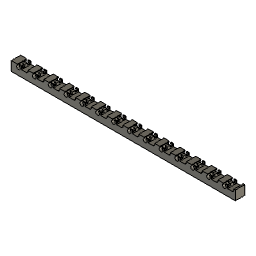
Assembly v11 (Autodesk Fusion 360 archive; units mm, degrees)
design "Pushing Bar"
Autodesk Fusion 360 part; units mm, degrees
sketch "Sketch1" plane through (0, 0, 0) normal (0, 0, 1) x (1, 0, 0)
  line L0 (390, 15) -> (-390, 15)
  line L1 (-390, 15) -> (-390, -15)
  line L2 (-390, -15) -> (390, -15)
  line L3 (390, -15) -> (390, 15)
  line L4 (390, 15) -> (-390, -15) construction
  line L5 (-390, 15) -> (390, -15) construction
  line L6 (3, -10) -> (-3, -10) construction
  line L7 (-3, -10) -> (-3, 10) construction
  line L8 (-3, 10) -> (3, 10) construction
  line L9 (3, 10) -> (3, -10) construction
  line L10 (3, -10) -> (-3, 10) construction
  line L11 (-3, -10) -> (3, 10) construction
  line L12 (-328.9372, 15) -> (390, 15)
  line L13 (390, 15) -> (390, -15)
  line L14 (390, -15) -> (-328.9372, -15)
  dimension "d2" = 780
  dimension "d5" = 20
  dimension "d6" = 6
  dimension "d7" = 5
  constraint horizontal L0
  constraint perpendicular L0 L1
  constraint parallel L0 L2
  constraint parallel L1 L3
  constraint coincident L4 origin
  constraint coincident L5 origin
  constraint horizontal L6
  constraint perpendicular L6 L7
  constraint parallel L6 L8
  constraint parallel L7 L9
  constraint coincident L10 origin
  constraint coincident L11 origin
  constraint horizontal L12
  constraint vertical L13
  constraint horizontal L14
  constraint coincident L0 L12.start
  measures "d2" distance of L0.start L0.end
  measures "d5" distance of L6.start L8.end
  measures "d6" distance of L7.end L8.end
  measures "d7" distance of L2 L6
extrude "Extrude1" add sketch "Sketch1" along normal mid plane 30
sketch "Sketch2" plane through (0, 0, 0) normal (0, 1, 0) x (1, 0, 0)
  circle A0 centre (339.2, -7.6834) radius 6 construction
  circle A1 centre (339.2, -11) radius 5
  line L0 (-390, -15) -> (390, -15)
  line L1 (334.2, -11) -> (344.2, -11) construction
  line L2 (390, -15) -> (390, 15) construction
  line L3 (342.2, -15) -> (336.2, -15)
  line L4 (336.2, -15) -> (336.2, -7)
  line L5 (336.2, -7) -> (342.2, -7)
  line L6 (342.2, -7) -> (342.2, -15)
  circle A2 centre (288.4, -11) radius 5
  circle A3 centre (237.6, -11) radius 5
  circle A4 centre (186.8, -11) radius 5
  circle A5 centre (136, -11) radius 5
  circle A6 centre (85.2, -11) radius 5
  circle A7 centre (34.4, -11) radius 5
  circle A8 centre (-16.4, -11) radius 5
  circle A9 centre (-67.2, -11) radius 5
  circle A10 centre (-118, -11) radius 5
  circle A11 centre (-168.8, -11) radius 5
  circle A12 centre (-219.6, -11) radius 5
  circle A13 centre (-270.4, -11) radius 5
  circle A14 centre (-321.2, -11) radius 5
  circle A15 centre (339.2, -12.3542) radius 4 construction
  dimension "d8" = 10
  dimension "d9" = 12
  dimension "d11" = 50.8
  dimension "d15" = 6
  dimension "d18" = -50.8
  dimension "d19" = 0
  dimension "d24" = 8
  constraint vertical A0.centre A1.centre
  constraint coincident A1 L1.start
  constraint coincident A1 L1.end
  constraint parallel L0 L1
  constraint coincident A1.centre L1
  constraint coincident A0 L1.start
  constraint horizontal L3
  constraint vertical L4
  constraint horizontal L5
  constraint vertical L6
  constraint coincident A1 L3.start
  constraint coincident L0 L3.start
  constraint coincident A1 L3.end
  constraint coincident A1 L5.end
  constraint coincident L3.end A15
  constraint coincident L3.start A15
  measures "d8" diameter of A1
  measures "d9" diameter of A0
  measures "d11" distance of A1.centre L2
  measures "d15" distance of L3.start L3.end
  measures "d24" diameter of A15
extrude "Extrude2" cut sketch "Sketch2" along normal mid plane 24 contours A1 L6 | A1 L5 | L0 L3 L4 L5 L6 | A1 L4 | L0 A14 | L0 A13 | L0 A12 | L0 A11 | L0 A10 | L0 A9 | L0 A8 | L0 A7 | L0 A6 | L0 A5 | L0 A4 | L0 A3 | L0 A2 picked at (-320.0174, -13.3398) picked at (-269.2174, -13.3398) picked at (-221.1787, -11.1742) picked at (-170.3787, -11.1742) picked at (-117.987, -11.8527) picked at (-66.8785, -11.7945) picked at (-17.7203, -12.3275) picked at (34.413, -11.8527) picked at (85.213, -11.8527) picked at (134.3807, -11.852) picked at (187.7455, -8.0418) picked at (238.5455, -8.0418) picked at (289.5826, -13.3398)
sketch "Sketch3" plane through (0, 0, 0) normal (0, 1, 0) x (1, 0, 0)
  circle A0 centre (339.2, -7.6834) radius 6
  line L0 (336.2, -15) -> (342.2, -15)
  line L1 (342.2, -12.8795) -> (342.2, -2.4872) construction
  line L2 (342.2, -2.4872) -> (336.2, -2.4872) construction
  line L3 (336.2, -2.4872) -> (336.2, -12.8795) construction
  circle A1 centre (339.2, -11) radius 5 construction
  line L4 (-390, -15) -> (390, -15)
  line L5 (342.2, -15) -> (342.2, -12.8795)
  line L6 (336.2, -12.8795) -> (336.2, -15)
  arc A2 (342.2, -12.8795) -> (336.2, -12.8795) centre (339.2, -7.6834) ccw
  arc A3 (336.2, -12.8795) -> (342.2, -12.8795) centre (339.2, -7.6834) ccw construction
  line L7 (285.4, -12.8795) -> (285.4, -15)
  line L8 (285.4, -15) -> (291.4, -15)
  arc A4 (291.4, -12.8795) -> (285.4, -12.8795) centre (288.4, -7.6834) ccw
  line L9 (291.4, -15) -> (291.4, -12.8795)
  line L10 (234.6, -12.8795) -> (234.6, -15)
  line L11 (234.6, -15) -> (240.6, -15)
  arc A5 (240.6, -12.8795) -> (234.6, -12.8795) centre (237.6, -7.6834) ccw
  line L12 (240.6, -15) -> (240.6, -12.8795)
  line L13 (183.8, -12.8795) -> (183.8, -15)
  line L14 (183.8, -15) -> (189.8, -15)
  arc A6 (189.8, -12.8795) -> (183.8, -12.8795) centre (186.8, -7.6834) ccw
  line L15 (189.8, -15) -> (189.8, -12.8795)
  line L16 (133, -12.8795) -> (133, -15)
  line L17 (133, -15) -> (139, -15)
  arc A7 (139, -12.8795) -> (133, -12.8795) centre (136, -7.6834) ccw
  line L18 (139, -15) -> (139, -12.8795)
  line L19 (82.2, -12.8795) -> (82.2, -15)
  line L20 (82.2, -15) -> (88.2, -15)
  arc A8 (88.2, -12.8795) -> (82.2, -12.8795) centre (85.2, -7.6834) ccw
  line L21 (88.2, -15) -> (88.2, -12.8795)
  line L22 (31.4, -12.8795) -> (31.4, -15)
  line L23 (31.4, -15) -> (37.4, -15)
  arc A9 (37.4, -12.8795) -> (31.4, -12.8795) centre (34.4, -7.6834) ccw
  line L24 (37.4, -15) -> (37.4, -12.8795)
  line L25 (-19.4, -12.8795) -> (-19.4, -15)
  line L26 (-19.4, -15) -> (-13.4, -15)
  arc A10 (-13.4, -12.8795) -> (-19.4, -12.8795) centre (-16.4, -7.6834) ccw
  line L27 (-13.4, -15) -> (-13.4, -12.8795)
  line L28 (-70.2, -12.8795) -> (-70.2, -15)
  line L29 (-70.2, -15) -> (-64.2, -15)
  arc A11 (-64.2, -12.8795) -> (-70.2, -12.8795) centre (-67.2, -7.6834) ccw
  line L30 (-64.2, -15) -> (-64.2, -12.8795)
  line L31 (-121, -12.8795) -> (-121, -15)
  line L32 (-121, -15) -> (-115, -15)
  arc A12 (-115, -12.8795) -> (-121, -12.8795) centre (-118, -7.6834) ccw
  line L33 (-115, -15) -> (-115, -12.8795)
  line L34 (-171.8, -12.8795) -> (-171.8, -15)
  line L35 (-171.8, -15) -> (-165.8, -15)
  arc A13 (-165.8, -12.8795) -> (-171.8, -12.8795) centre (-168.8, -7.6834) ccw
  line L36 (-165.8, -15) -> (-165.8, -12.8795)
  line L37 (-222.6, -12.8795) -> (-222.6, -15)
  line L38 (-222.6, -15) -> (-216.6, -15)
  arc A14 (-216.6, -12.8795) -> (-222.6, -12.8795) centre (-219.6, -7.6834) ccw
  line L39 (-216.6, -15) -> (-216.6, -12.8795)
  line L40 (-273.4, -12.8795) -> (-273.4, -15)
  line L41 (-273.4, -15) -> (-267.4, -15)
  arc A15 (-267.4, -12.8795) -> (-273.4, -12.8795) centre (-270.4, -7.6834) ccw
  line L42 (-267.4, -15) -> (-267.4, -12.8795)
  line L43 (-324.2, -12.8795) -> (-324.2, -15)
  line L44 (-324.2, -15) -> (-318.2, -15)
  arc A16 (-318.2, -12.8795) -> (-324.2, -12.8795) centre (-321.2, -7.6834) ccw
  line L45 (-318.2, -15) -> (-318.2, -12.8795)
  dimension "d22" = -50.8
  dimension "d23" = 0
  constraint equal A0 A2
  constraint horizontal L0
  constraint vertical L1
  constraint horizontal L2
  constraint vertical L3
  constraint coincident L0.start A1
  constraint coincident L0.end A1
  constraint coincident L0.end L4
  constraint coincident L2.end A2
  constraint coincident A0.centre A2.centre
  constraint vertical L5
  constraint vertical L6
  constraint concentric A2 A3
extrude "Extrude3" cut sketch "Sketch3" along normal through all and the other way through all
sketch "Sketch4" plane through (0, 0, 0) normal (0, 1, 0) x (1, 0, 0)
  line L0 (339.2, -9.5) -> (341.7981, -9.5) construction
  line L1 (349.2, -9.5) -> (349.2, -12.5) construction
  line L2 (341.7981, -12.5) -> (339.2, -12.5) construction
  line L3 (339.2, -12.5) -> (339.2, -9.5) construction
  line L4 (349.2, -6) -> (364.819, -6)
  line L5 (364.819, -6) -> (364.819, -16) construction
  line L6 (364.819, -16) -> (341.7981, -16)
  line L7 (349.2, -12.5) -> (349.2, -9.5) construction
  line L8 (349.2, -9.5) -> (349.2, -6)
  arc A0 (364.819, -16) -> (364.819, -6) centre (364.819, -11) ccw
  arc A1 (364.819, -6) -> (364.819, -16) centre (364.819, -11) ccw construction
  line L9 (341.7981, -9.5) -> (349.2, -9.5)
  arc A2 (341.7981, -9.5) -> (341.7981, -12.5) centre (339.2, -11) ccw construction
  line L10 (341.7981, -16) -> (341.7981, -9.5)
  line L11 (349.2, -6) -> (364.819, -6)
  line L12 (364.819, -16) -> (349.2, -16)
  line L13 (349.2, -16) -> (349.2, -6)
  line L14 (349.2, -16) -> (349.2, -6)
  arc A3 (314.019, -16) -> (314.019, -6) centre (314.019, -11) ccw
  line L15 (314.019, -16) -> (298.4, -16)
  line L16 (314.019, -16) -> (290.9981, -16)
  line L17 (290.9981, -16) -> (290.9981, -9.5)
  line L18 (290.9981, -9.5) -> (298.4, -9.5)
  line L19 (298.4, -9.5) -> (298.4, -6)
  line L20 (298.4, -6) -> (314.019, -6)
  arc A4 (263.219, -16) -> (263.219, -6) centre (263.219, -11) ccw
  line L21 (263.219, -16) -> (247.6, -16)
  line L22 (263.219, -16) -> (240.1981, -16)
  line L23 (240.1981, -16) -> (240.1981, -9.5)
  line L24 (240.1981, -9.5) -> (247.6, -9.5)
  line L25 (247.6, -9.5) -> (247.6, -6)
  line L26 (247.6, -6) -> (263.219, -6)
  arc A5 (212.419, -16) -> (212.419, -6) centre (212.419, -11) ccw
  line L27 (212.419, -16) -> (196.8, -16)
  line L28 (212.419, -16) -> (189.3981, -16)
  line L29 (189.3981, -16) -> (189.3981, -9.5)
  line L30 (189.3981, -9.5) -> (196.8, -9.5)
  line L31 (196.8, -9.5) -> (196.8, -6)
  line L32 (196.8, -6) -> (212.419, -6)
  arc A6 (161.619, -16) -> (161.619, -6) centre (161.619, -11) ccw
  line L33 (161.619, -16) -> (146, -16)
  line L34 (161.619, -16) -> (138.5981, -16)
  line L35 (138.5981, -16) -> (138.5981, -9.5)
  line L36 (138.5981, -9.5) -> (146, -9.5)
  line L37 (146, -9.5) -> (146, -6)
  line L38 (146, -6) -> (161.619, -6)
  arc A7 (110.819, -16) -> (110.819, -6) centre (110.819, -11) ccw
  line L39 (110.819, -16) -> (95.2, -16)
  line L40 (110.819, -16) -> (87.7981, -16)
  line L41 (87.7981, -16) -> (87.7981, -9.5)
  line L42 (87.7981, -9.5) -> (95.2, -9.5)
  line L43 (95.2, -9.5) -> (95.2, -6)
  line L44 (95.2, -6) -> (110.819, -6)
  arc A8 (60.019, -16) -> (60.019, -6) centre (60.019, -11) ccw
  line L45 (60.019, -16) -> (44.4, -16)
  line L46 (60.019, -16) -> (36.9981, -16)
  line L47 (36.9981, -16) -> (36.9981, -9.5)
  line L48 (36.9981, -9.5) -> (44.4, -9.5)
  line L49 (44.4, -9.5) -> (44.4, -6)
  line L50 (44.4, -6) -> (60.019, -6)
  arc A9 (9.219, -16) -> (9.219, -6) centre (9.219, -11) ccw
  line L51 (9.219, -16) -> (-6.4, -16)
  line L52 (9.219, -16) -> (-13.8019, -16)
  line L53 (-13.8019, -16) -> (-13.8019, -9.5)
  line L54 (-13.8019, -9.5) -> (-6.4, -9.5)
  line L55 (-6.4, -9.5) -> (-6.4, -6)
  line L56 (-6.4, -6) -> (9.219, -6)
  arc A10 (-41.581, -16) -> (-41.581, -6) centre (-41.581, -11) ccw
  line L57 (-41.581, -16) -> (-57.2, -16)
  line L58 (-41.581, -16) -> (-64.6019, -16)
  line L59 (-64.6019, -16) -> (-64.6019, -9.5)
  line L60 (-64.6019, -9.5) -> (-57.2, -9.5)
  line L61 (-57.2, -9.5) -> (-57.2, -6)
  line L62 (-57.2, -6) -> (-41.581, -6)
  arc A11 (-92.381, -16) -> (-92.381, -6) centre (-92.381, -11) ccw
  line L63 (-92.381, -16) -> (-108, -16)
  line L64 (-92.381, -16) -> (-115.4019, -16)
  line L65 (-115.4019, -16) -> (-115.4019, -9.5)
  line L66 (-115.4019, -9.5) -> (-108, -9.5)
  line L67 (-108, -9.5) -> (-108, -6)
  line L68 (-108, -6) -> (-92.381, -6)
  arc A12 (-143.181, -16) -> (-143.181, -6) centre (-143.181, -11) ccw
  line L69 (-143.181, -16) -> (-158.8, -16)
  line L70 (-143.181, -16) -> (-166.2019, -16)
  line L71 (-166.2019, -16) -> (-166.2019, -9.5)
  line L72 (-166.2019, -9.5) -> (-158.8, -9.5)
  line L73 (-158.8, -9.5) -> (-158.8, -6)
  line L74 (-158.8, -6) -> (-143.181, -6)
  arc A13 (-193.981, -16) -> (-193.981, -6) centre (-193.981, -11) ccw
  line L75 (-193.981, -16) -> (-209.6, -16)
  line L76 (-193.981, -16) -> (-217.0019, -16)
  line L77 (-217.0019, -16) -> (-217.0019, -9.5)
  line L78 (-217.0019, -9.5) -> (-209.6, -9.5)
  line L79 (-209.6, -9.5) -> (-209.6, -6)
  line L80 (-209.6, -6) -> (-193.981, -6)
  arc A14 (-244.781, -16) -> (-244.781, -6) centre (-244.781, -11) ccw
  line L81 (-244.781, -16) -> (-260.4, -16)
  line L82 (-244.781, -16) -> (-267.8019, -16)
  line L83 (-267.8019, -16) -> (-267.8019, -9.5)
  line L84 (-267.8019, -9.5) -> (-260.4, -9.5)
  line L85 (-260.4, -9.5) -> (-260.4, -6)
  line L86 (-260.4, -6) -> (-244.781, -6)
  arc A15 (-295.581, -16) -> (-295.581, -6) centre (-295.581, -11) ccw
  line L87 (-295.581, -16) -> (-311.2, -16)
  line L88 (-295.581, -16) -> (-318.6019, -16)
  line L89 (-318.6019, -16) -> (-318.6019, -9.5)
  line L90 (-318.6019, -9.5) -> (-311.2, -9.5)
  line L91 (-311.2, -9.5) -> (-311.2, -6)
  line L92 (-311.2, -6) -> (-295.581, -6)
  point P0 (339.2, -11)
  point P1 (349.2, -11)
  dimension "d25" = 6
  dimension "d26" = 3
  dimension "d27" = 10
  dimension "d29" = 15.619
  dimension "d31" = 3.5
  dimension "d32" = 5
  dimension "d43" = -50.8
  dimension "d44" = 0
  constraint coincident P0 A2.centre
  constraint horizontal L0
  constraint vertical L1
  constraint horizontal L2
  constraint vertical L3
  constraint coincident P0 L3
  constraint midpoint P0 L3
  constraint horizontal L4
  constraint vertical L5
  constraint horizontal L6
  constraint vertical L7
  constraint collinear L1 L7
  constraint coincident L7 P1
  constraint midpoint L1 P1
  constraint midpoint L5 A0.centre
  constraint concentric A0 A1
  constraint horizontal L9
  constraint vertical L8
  constraint vertical L10
  constraint horizontal L11
  constraint horizontal L12
  constraint vertical L13
  constraint vertical L14
  measures "d25" diameter of A2
  measures "d26" distance of L0 L2
  measures "d27" distance of P0 L1
  measures "d29" distance of L4.start L4.end
  measures "d31" distance of L1.start L4.start
  measures "d32" radius of A1
extrude "Extrude4" cut sketch "Sketch4" along normal blind 7 from surface at 5
extrude "Extrude5" cut sketch "Sketch4" against normal blind 7 from surface at -5
extrude "Extrude6" cut sketch "Sketch4" along normal through all and the other way through all contours L4 L6 L8 A0 L11 L12 L13 L14
sketch "Sketch5" plane through (0, 0, 0) normal (0, 1, 0) x (1, 0, 0)
  line L0 (349.2, -16) -> (369.819, -16)
  line L1 (369.819, -16) -> (369.819, -11)
  line L2 (364.819, -6) -> (349.2, -6)
  line L3 (349.2, -6) -> (349.2, -16)
  arc A0 (364.819, -16) -> (364.819, -6) centre (364.819, -11) ccw
  arc A1 (369.819, -11) -> (364.819, -6) centre (364.819, -11) ccw
  line L4 (369.819, -6) -> (364.819, -6) construction
  line L5 (369.819, -11) -> (369.819, -6) construction
  line L6 (298.4, -16) -> (319.019, -16)
  line L7 (298.4, -6) -> (298.4, -16)
  line L8 (314.019, -6) -> (298.4, -6)
  arc A2 (319.019, -11) -> (314.019, -6) centre (314.019, -11) ccw
  line L9 (319.019, -16) -> (319.019, -11)
  line L10 (247.6, -16) -> (268.219, -16)
  line L11 (247.6, -6) -> (247.6, -16)
  line L12 (263.219, -6) -> (247.6, -6)
  arc A3 (268.219, -11) -> (263.219, -6) centre (263.219, -11) ccw
  line L13 (268.219, -16) -> (268.219, -11)
  line L14 (196.8, -16) -> (217.419, -16)
  line L15 (196.8, -6) -> (196.8, -16)
  line L16 (212.419, -6) -> (196.8, -6)
  arc A4 (217.419, -11) -> (212.419, -6) centre (212.419, -11) ccw
  line L17 (217.419, -16) -> (217.419, -11)
  line L18 (146, -16) -> (166.619, -16)
  line L19 (146, -6) -> (146, -16)
  line L20 (161.619, -6) -> (146, -6)
  arc A5 (166.619, -11) -> (161.619, -6) centre (161.619, -11) ccw
  line L21 (166.619, -16) -> (166.619, -11)
  line L22 (95.2, -16) -> (115.819, -16)
  line L23 (95.2, -6) -> (95.2, -16)
  line L24 (110.819, -6) -> (95.2, -6)
  arc A6 (115.819, -11) -> (110.819, -6) centre (110.819, -11) ccw
  line L25 (115.819, -16) -> (115.819, -11)
  line L26 (44.4, -16) -> (65.019, -16)
  line L27 (44.4, -6) -> (44.4, -16)
  line L28 (60.019, -6) -> (44.4, -6)
  arc A7 (65.019, -11) -> (60.019, -6) centre (60.019, -11) ccw
  line L29 (65.019, -16) -> (65.019, -11)
  line L30 (-6.4, -16) -> (14.219, -16)
  line L31 (-6.4, -6) -> (-6.4, -16)
  line L32 (9.219, -6) -> (-6.4, -6)
  arc A8 (14.219, -11) -> (9.219, -6) centre (9.219, -11) ccw
  line L33 (14.219, -16) -> (14.219, -11)
  line L34 (-57.2, -16) -> (-36.581, -16)
  line L35 (-57.2, -6) -> (-57.2, -16)
  line L36 (-41.581, -6) -> (-57.2, -6)
  arc A9 (-36.581, -11) -> (-41.581, -6) centre (-41.581, -11) ccw
  line L37 (-36.581, -16) -> (-36.581, -11)
  line L38 (-108, -16) -> (-87.381, -16)
  line L39 (-108, -6) -> (-108, -16)
  line L40 (-92.381, -6) -> (-108, -6)
  arc A10 (-87.381, -11) -> (-92.381, -6) centre (-92.381, -11) ccw
  line L41 (-87.381, -16) -> (-87.381, -11)
  line L42 (-158.8, -16) -> (-138.181, -16)
  line L43 (-158.8, -6) -> (-158.8, -16)
  line L44 (-143.181, -6) -> (-158.8, -6)
  arc A11 (-138.181, -11) -> (-143.181, -6) centre (-143.181, -11) ccw
  line L45 (-138.181, -16) -> (-138.181, -11)
  line L46 (-209.6, -16) -> (-188.981, -16)
  line L47 (-209.6, -6) -> (-209.6, -16)
  line L48 (-193.981, -6) -> (-209.6, -6)
  arc A12 (-188.981, -11) -> (-193.981, -6) centre (-193.981, -11) ccw
  line L49 (-188.981, -16) -> (-188.981, -11)
  line L50 (-260.4, -16) -> (-239.781, -16)
  line L51 (-260.4, -6) -> (-260.4, -16)
  line L52 (-244.781, -6) -> (-260.4, -6)
  arc A13 (-239.781, -11) -> (-244.781, -6) centre (-244.781, -11) ccw
  line L53 (-239.781, -16) -> (-239.781, -11)
  line L54 (-311.2, -16) -> (-290.581, -16)
  line L55 (-311.2, -6) -> (-311.2, -16)
  line L56 (-295.581, -6) -> (-311.2, -6)
  arc A14 (-290.581, -11) -> (-295.581, -6) centre (-295.581, -11) ccw
  line L57 (-290.581, -16) -> (-290.581, -11)
  point P0 (349.2, -16)
  dimension "d47" = -50.8
  dimension "d48" = 0
  constraint horizontal L0
  constraint vertical L1
  constraint horizontal L2
  constraint vertical L3
  constraint tangent L1 A0
  constraint tangent L0 A0
  constraint tangent L2 A0
  constraint coincident L3 P0
  constraint coincident L2.start A0.end
  constraint midpoint A0 L1.end
extrude "Extrude7" cut sketch "Sketch5" along normal through all and the other way through all
sketch "Sketch6" plane through (0, 0, 15) normal (0, 0, 1) x (-1, 0, 0)
  line L0 (324.2, 15) -> (324.2, 12)
  line L1 (324.2, 12) -> (324.2, -12)
  line L2 (324.2, -12) -> (324.2, -15)
  line L3 (324.2, -15) -> (390, -15)
  line L4 (390, -15) -> (390, 15)
  line L5 (390, 15) -> (324.2, 15)
  line L6 (390, 15) -> (344.2, 15)
  line L7 (344.2, 15) -> (344.2, -15)
  line L8 (344.2, -15) -> (390, -15)
  line L9 (390, -15) -> (390, 15)
  line L10 (-390, -15) -> (-374.819, -15)
  line L11 (-374.819, -15) -> (-374.819, 15)
  line L12 (-374.819, 15) -> (-390, 15)
  line L13 (-390, 15) -> (-390, -15)
  line L14 (-390, -15) -> (-369.819, -15)
  line L15 (-369.819, 15) -> (-390, 15)
  line L16 (-390, 15) -> (-390, -15)
  line L17 (-369.819, -15) -> (-369.819, 15)
  dimension "d50" = 20
  dimension "d52" = 5
  constraint horizontal L6
  constraint vertical L7
  constraint horizontal L8
  constraint vertical L9
  constraint coincident L3 L7.end
  constraint coincident L4.end L5.start
  constraint horizontal L10
  constraint vertical L11
  constraint horizontal L12
  constraint vertical L13
  constraint collinear L10 L14
  constraint collinear L12 L15
  constraint collinear L13 L16
  measures "d50" distance of L1 L7
  measures "d52" distance of L11 L17
extrude "Extrude8" cut sketch "Sketch6" against normal through all contours L3 L4 L5 L6 L7 L8 L9 | L10 L11 L12 L13 L14 L15 L16
equation "d8 = 8 mm + 2 mm"
equation "d11 = ( 25.4 * 2 ) * 1 mm"
equation "d18 = ( -25.4 * 2 ) * 1 mm"
equation "d43 = ( -25.4 * 2 ) * 1 mm"
equation "d47 = ( -25.4 * 2 ) * 1 mm"

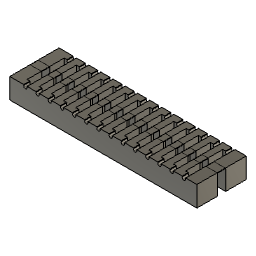
design "Grate Bars"
Autodesk Fusion 360 part; units mm, degrees
sketch "Sketch1" plane through (0, 0, 0) normal (0, 0, 1) x (1, 0, 0)
  line L0 (390, -102.9) -> (-390, -102.9)
  line L1 (-390, -102.9) -> (-390, 102.9)
  line L2 (-390, 102.9) -> (390, 102.9)
  line L3 (390, 102.9) -> (390, -102.9)
  line L4 (390, -102.9) -> (-390, 102.9) construction
  line L5 (-390, -102.9) -> (390, 102.9) construction
  dimension "d1" = 780
  dimension "d2" = 205.8
  constraint horizontal L0
  constraint perpendicular L0 L1
  constraint parallel L0 L2
  constraint parallel L1 L3
  constraint coincident L4 origin
  constraint coincident L5 origin
  measures "d1" distance of L1.end L2.end
  measures "d2" distance of L0.start L2.end
extrude "Extrude1" add sketch "Sketch1" along normal mid plane 85
sketch "Sketch2" plane through (0, 0, 42.5) normal (0, 0, 1) x (-1, 0, 0)
  line L0 (-390, -102.9) -> (390, -102.9)
  line L1 (390, -102.9) -> (390, 102.9)
  line L2 (390, 102.9) -> (-390, 102.9)
  line L3 (-390, 102.9) -> (-390, -102.9)
  line L4 (317.5, 77.5) -> (342.9, 77.5)
  line L5 (342.9, 77.5) -> (342.9, -77.5)
  line L6 (342.9, -77.5) -> (317.5, -77.5)
  line L7 (317.5, -77.5) -> (317.5, 77.5)
  line L8 (317.5, 77.5) -> (342.9, -77.5) construction
  line L9 (342.9, 77.5) -> (317.5, -77.5) construction
  line L10 (292.1, 77.5) -> (292.1, -77.5)
  line L11 (292.1, -77.5) -> (266.7, -77.5)
  line L12 (266.7, -77.5) -> (266.7, 77.5)
  line L13 (266.7, 77.5) -> (292.1, 77.5)
  line L14 (241.3, 77.5) -> (241.3, -77.5)
  line L15 (241.3, -77.5) -> (215.9, -77.5)
  line L16 (215.9, -77.5) -> (215.9, 77.5)
  line L17 (215.9, 77.5) -> (241.3, 77.5)
  line L18 (190.5, 77.5) -> (190.5, -77.5)
  line L19 (190.5, -77.5) -> (165.1, -77.5)
  line L20 (165.1, -77.5) -> (165.1, 77.5)
  line L21 (165.1, 77.5) -> (190.5, 77.5)
  line L22 (139.7, 77.5) -> (139.7, -77.5)
  line L23 (139.7, -77.5) -> (114.3, -77.5)
  line L24 (114.3, -77.5) -> (114.3, 77.5)
  line L25 (114.3, 77.5) -> (139.7, 77.5)
  line L26 (88.9, 77.5) -> (88.9, -77.5)
  line L27 (88.9, -77.5) -> (63.5, -77.5)
  line L28 (63.5, -77.5) -> (63.5, 77.5)
  line L29 (63.5, 77.5) -> (88.9, 77.5)
  line L30 (38.1, 77.5) -> (38.1, -77.5)
  line L31 (38.1, -77.5) -> (12.7, -77.5)
  line L32 (12.7, -77.5) -> (12.7, 77.5)
  line L33 (12.7, 77.5) -> (38.1, 77.5)
  line L34 (-12.7, 77.5) -> (-12.7, -77.5)
  line L35 (-12.7, -77.5) -> (-38.1, -77.5)
  line L36 (-38.1, -77.5) -> (-38.1, 77.5)
  line L37 (-38.1, 77.5) -> (-12.7, 77.5)
  line L38 (-63.5, 77.5) -> (-63.5, -77.5)
  line L39 (-63.5, -77.5) -> (-88.9, -77.5)
  line L40 (-88.9, -77.5) -> (-88.9, 77.5)
  line L41 (-88.9, 77.5) -> (-63.5, 77.5)
  line L42 (-114.3, 77.5) -> (-114.3, -77.5)
  line L43 (-114.3, -77.5) -> (-139.7, -77.5)
  line L44 (-139.7, -77.5) -> (-139.7, 77.5)
  line L45 (-139.7, 77.5) -> (-114.3, 77.5)
  line L46 (-165.1, 77.5) -> (-165.1, -77.5)
  line L47 (-165.1, -77.5) -> (-190.5, -77.5)
  line L48 (-190.5, -77.5) -> (-190.5, 77.5)
  line L49 (-190.5, 77.5) -> (-165.1, 77.5)
  line L50 (-215.9, 77.5) -> (-215.9, -77.5)
  line L51 (-215.9, -77.5) -> (-241.3, -77.5)
  line L52 (-241.3, -77.5) -> (-241.3, 77.5)
  line L53 (-241.3, 77.5) -> (-215.9, 77.5)
  line L54 (-266.7, 77.5) -> (-266.7, -77.5)
  line L55 (-266.7, -77.5) -> (-292.1, -77.5)
  line L56 (-292.1, -77.5) -> (-292.1, 77.5)
  line L57 (-292.1, 77.5) -> (-266.7, 77.5)
  line L58 (-317.5, 77.5) -> (-317.5, -77.5)
  line L59 (-317.5, -77.5) -> (-342.9, -77.5)
  line L60 (-342.9, -77.5) -> (-342.9, 77.5)
  line L61 (-342.9, 77.5) -> (-317.5, 77.5)
  point P0 (330.2, 0)
  dimension "d5" = 25.4
  dimension "d7" = 25.4
  dimension "d10" = -50.8
  dimension "d11" = 0
  dimension "d14" = 47.1
  constraint horizontal L4
  constraint perpendicular L4 L5
  constraint parallel L4 L6
  constraint parallel L5 L7
  constraint coincident L8 P0
  constraint coincident L9 P0
  constraint horizontal origin P0
  measures "d5" distance of L0 L6
  measures "d7" distance of L4.start L4.end
  measures "d14" distance of L1 L5
extrude "Extrude2" cut sketch "Sketch2" against normal up to surface (85 mm away) contours L4 L5 L6 L7 | L10 L11 L12 L13 | L14 L15 L16 L17 | L18 L19 L20 L21 | L22 L23 L24 L25 | L26 L27 L28 L29 | L30 L31 L32 L33 | L34 L35 L36 L37 | L38 L39 L40 L41 | L42 L43 L44 L45 | L46 L47 L48 L49 | L50 L51 L52 L53 | L54 L55 L56 L57 | L58 L59 L60 L61
sketch "Sketch3" plane through (0, 0, 0) normal (0, 1, 0) x (1, 0, 0)
  circle A0 centre (335.9, -37.5) radius 7
  line L0 (317.5, -42.5) -> (317.5, 42.5)
  line L1 (390, -42.5) -> (-390, -42.5)
  line L2 (342.9, -42.5) -> (342.9, 42.5)
  circle A1 centre (285.1, -37.5) radius 7
  circle A2 centre (234.3, -37.5) radius 7
  circle A3 centre (183.5, -37.5) radius 7
  circle A4 centre (132.7, -37.5) radius 7
  circle A5 centre (81.9, -37.5) radius 7
  circle A6 centre (31.1, -37.5) radius 7
  circle A7 centre (-19.7, -37.5) radius 7
  circle A8 centre (-70.5, -37.5) radius 7
  circle A9 centre (-121.3, -37.5) radius 7
  circle A10 centre (-172.1, -37.5) radius 7
  circle A11 centre (-222.9, -37.5) radius 7
  circle A12 centre (-273.7, -37.5) radius 7
  circle A13 centre (-324.5, -37.5) radius 7
  dimension "d19" = 14
  dimension "d23" = 7
  dimension "d24" = 5
  dimension "d27" = -50.8
  dimension "d28" = 0
  measures "d19" diameter of A0
  measures "d23" distance of A0.centre L2
  measures "d24" distance of A0.centre L1
extrude "Extrude3" cut sketch "Sketch3" along normal through all and the other way through all contours A0 L1 | L1 A1 | L1 A2 | L1 A3 | L1 A4 | L1 A5 | L1 A6 | L1 A7 | L1 A8 | L1 A9 | L1 A10 | L1 A11 | L1 A12 | L1 A13 picked at (338.1343, -37.5876) picked at (287.3343, -37.5876) picked at (232.5837, -36.5434) picked at (181.7837, -36.5434) picked at (131.458, -35.7084) picked at (83.3358, -37.9253) picked at (29.0436, -38.7503) picked at (-18.0005, -40.5961) picked at (-69.9038, -38.5775) picked at (-120.1856, -37.8147) picked at (-170.3604, -35.9462) picked at (-220.8946, -36.7332) picked at (-271.4657, -37.5876) picked at (-322.2657, -37.5876)
fillet "Fillet1" radius 1 8 edges at (340.799, -90.2, 42.5) (331.001, -90.2, 42.5) (340.799, 90.2, 42.5) (331.001, 90.2, 42.5) (289.999, -90.2, 42.5) (280.201, -90.2, 42.5) (289.999, 90.2, 42.5) (280.201, 90.2, 42.5)
fillet "Fillet1" radius 1 48 edges at (229.401, 90.2, 42.5) (239.199, 90.2, 42.5) (229.401, -90.2, 42.5) (239.199, -90.2, 42.5) (188.399, -90.2, 42.5) (178.601, -90.2, 42.5) (188.399, 90.2, 42.5) (178.601, 90.2, 42.5) (137.599, 90.2, 42.5) (127.801, 90.2, 42.5) (137.599, -90.2, 42.5) (127.801, -90.2, 42.5) (86.799, -90.2, 42.5) (77.001, -90.2, 42.5) (86.799, 90.2, 42.5) (77.001, 90.2, 42.5) (35.999, 90.2, 42.5) (26.201, 90.2, 42.5) (35.999, -90.2, 42.5) (26.201, -90.2, 42.5) (-14.801, -90.2, 42.5) (-24.599, -90.2, 42.5) (-14.801, 90.2, 42.5) (-24.599, 90.2, 42.5) (-65.601, 90.2, 42.5) (-75.399, 90.2, 42.5) (-65.601, -90.2, 42.5) (-75.399, -90.2, 42.5) (-116.401, -90.2, 42.5) (-126.199, -90.2, 42.5) (-116.401, 90.2, 42.5) (-126.199, 90.2, 42.5) (-167.201, 90.2, 42.5) (-176.999, 90.2, 42.5) (-167.201, -90.2, 42.5) (-176.999, -90.2, 42.5) (-218.001, -90.2, 42.5) (-227.799, -90.2, 42.5) (-218.001, 90.2, 42.5) (-227.799, 90.2, 42.5) (-268.801, 90.2, 42.5) (-278.599, 90.2, 42.5) (-278.599, -90.2, 42.5) (-268.801, -90.2, 42.5) (-329.399, -90.2, 42.5) (-319.601, -90.2, 42.5) (-319.601, 90.2, 42.5) (-329.399, 90.2, 42.5)
sketch "Sketch4" plane through (390, 0, 0) normal (1, 0, 0) x (0, 1, 0)
  line L0 (102.9, -42.5) -> (102.9, 42.5)
  line L1 (102.9, 42.5) -> (-102.9, 42.5)
  line L2 (-102.9, 42.5) -> (-102.9, -42.5)
  line L3 (-102.9, -42.5) -> (102.9, -42.5)
  line L4 (-17, -42.5) -> (17, -42.5)
  line L5 (17, -42.5) -> (17, 40.5)
  line L6 (17, 40.5) -> (-17, 40.5)
  line L7 (-17, 40.5) -> (-17, -42.5)
  line L8 (-17, 40.5) -> (17, -42.5) construction
  line L9 (17, 40.5) -> (-17, -42.5) construction
  line L10 (0, 40.5) -> (0, -42.5) construction
  point P0 (0, -1)
  dimension "d34" = 17
  dimension "d36" = 2
  constraint horizontal L4
  constraint vertical L5
  constraint horizontal L6
  constraint vertical L7
  constraint coincident L3 L4.start
  constraint midpoint L9 P0
  constraint coincident L6 L10.start
  constraint coincident L3 L10.end
  constraint vertical L10
  constraint coincident origin L10
  constraint vertical origin P0
  measures "d34" distance of L7 L10
  measures "d36" distance of L1 L6
extrude "Extrude4" cut sketch "Sketch4" along normal through all and the other way through all contours L3 L4 L5 L6 L7
sketch "Sketch5" plane through (390, 0, 0) normal (1, 0, 0) x (0, 1, 0)
  line L0 (-17, -42.5) -> (-17, 40.5)
  line L1 (-17, 40.5) -> (17, 40.5)
  line L2 (17, 40.5) -> (17, -42.5)
  line L3 (17, -42.5) -> (102.9, -42.5)
  line L4 (102.9, -42.5) -> (102.9, 42.5)
  line L5 (102.9, 42.5) -> (-102.9, 42.5)
  line L6 (-102.9, 42.5) -> (-102.9, -42.5)
  line L7 (-102.9, -42.5) -> (-17, -42.5)
  line L8 (-21.5, 40.5) -> (21.5, 40.5)
  line L9 (21.5, 40.5) -> (21.5, -2.5)
  line L10 (21.5, -2.5) -> (-21.5, -2.5)
  line L11 (-21.5, -2.5) -> (-21.5, 40.5)
  point P0 (0, 40.5)
  point P1 (0, 40.5)
  dimension "d38" = 43
  dimension "d39" = 43
  constraint horizontal L8
  constraint vertical L9
  constraint horizontal L10
  constraint vertical L11
  constraint midpoint L1 P1
  constraint midpoint L8 P1
  constraint coincident P1 P0
  measures "d38" distance of L8.end L9.end
  measures "d39" distance of L8.start L8.end
equation "d2 = 155 mm + ( 25.4 * 2 ) * 1 mm"
equation "d14 = ( 780 mm - ( ( 27 * 25.4 ) * 1 mm ) ) / 2"
equation "d19 = 10 mm + 4 mm"
equation "d27 = ( -25.4 * 2 ) * 1 mm"

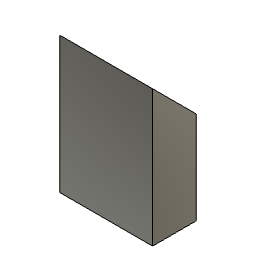
design "Slanted Block"
Autodesk Fusion 360 part; units mm, degrees
sketch "Sketch1" plane through (0, 0, 0) normal (0, 0, 1) x (1, 0, 0)
  line L0 (17, -8) -> (-17, -8)
  line L1 (-17, -8) -> (-17, 8)
  line L2 (-17, 8) -> (17, 8)
  line L3 (17, 8) -> (17, -8)
  line L4 (17, -8) -> (-17, 8) construction
  line L5 (-17, -8) -> (17, 8) construction
  circle A0 centre (0, 0) radius 5.831
  dimension "d1" = 11.662
  dimension "d2" = 34
  dimension "d3" = 16
  constraint horizontal L0
  constraint perpendicular L0 L1
  constraint parallel L0 L2
  constraint parallel L1 L3
  constraint coincident L4 A0.centre
  constraint coincident L5 A0.centre
  constraint coincident A0.centre origin
  measures "d1" diameter of A0
  measures "d2" distance of L1.end L2.end
  measures "d3" distance of L0.start L2.end
extrude "Extrude1" add sketch "Sketch1" along normal mid plane 50
ref_plane "WorkPlane1" through (0, -8, 15) normal (0, 0.707107, 0.707107) x (-1, 0, 0)
sketch "Sketch3" plane through (0, -8, 15) normal (0, 0.707107, 0.707107) x (-1, 0, 0)
  line L0 (17, 7.0711) -> (-17, 7.0711)
  line L1 (-17, 7.0711) -> (-17, -27.9289)
  line L2 (-17, -27.9289) -> (17, -27.9289)
  line L3 (17, -27.9289) -> (17, 7.0711)
  line L4 (17, 7.0711) -> (-17, 7.0711)
  line L5 (-17, -28.2843) -> (17, -28.2843)
  line L6 (-17, -28.2843) -> (-17, 7.0711)
  line L7 (17, -28.2843) -> (17, 7.0711)
  dimension "d8" = 35
  constraint horizontal L0
  constraint vertical L1
  constraint horizontal L2
  constraint vertical L3
  constraint collinear L0 L4
  constraint collinear L1 L6
  constraint collinear L3 L7
  measures "d8" distance of L0 L2
extrude "Extrude2" cut sketch "Sketch3" along normal through all from surface at 7
equation "d1 = ( 5.831 * 2 ) * 1 mm"

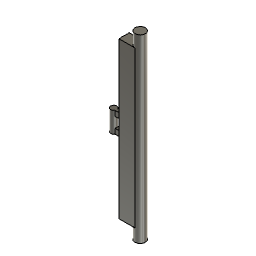
design "Slot (better)"
Autodesk Fusion 360 part; units mm, degrees
sketch "Sketch1" plane through (0, 0, 0) normal (0, 0, 1) x (1, 0, 0)
  line L0 (0, 0) -> (25.4, 0) construction
  line L1 (25.4, 0) -> (25.4, 50) construction
  line L2 (25.4, 50) -> (0, 50) construction
  line L3 (0, 50) -> (0, 0) construction
  line L4 (-7, 40) -> (-22.6192, 40)
  line L5 (-22.6192, 40) -> (-22.6192, 50)
  line L6 (-22.6192, 50) -> (-7, 50)
  line L7 (-7, 50) -> (-7, 40)
  circle A0 centre (-7, 45) radius 7 construction
  line L8 (0, 50) -> (-12.1416, 50) construction
  line L9 (-7, 45) -> (-22.6192, 45) construction
  line L10 (-25.4, 0) -> (-50.8, 0) construction
  line L11 (-50.8, 0) -> (-50.8, 50) construction
  line L12 (-50.8, 50) -> (-25.4, 50) construction
  line L13 (-25.4, 50) -> (-25.4, 0) construction
  circle A1 centre (-7, 45) radius 16.4 construction
  circle A2 centre (-7, 45) radius 18.4 construction
  arc A3 (-7, 40) -> (-7, 50) centre (-7, 45) ccw
  arc A4 (-7, 50) -> (-12, 45) centre (-7, 45) ccw construction
  arc A5 (-12, 45) -> (-7, 40) centre (-7, 45) ccw construction
  point P0 (-7, 45)
  dimension "d1" = 50
  dimension "d2" = 25.4
  dimension "d4" = 10
  dimension "d6" = 25.4
  dimension "d9" = 2
  dimension "d14" = 2
  constraint horizontal L0
  constraint vertical L1
  constraint horizontal L2
  constraint vertical L3
  constraint coincident L0.start L3.end
  constraint perpendicular L4 L5
  constraint parallel L4 L6
  constraint parallel L5 L7
  constraint coincident P0 A0.centre
  constraint concentric A0 A3
  constraint midpoint L7 P0
  constraint perpendicular L3 L8
  constraint tangent L8 A3
  constraint midpoint L5 L9.end
  constraint horizontal L10
  constraint vertical L11
  constraint horizontal L12
  constraint vertical L13
  constraint equal L2 L12
  constraint equal L3 L13
  constraint collinear L0 L10
  constraint coincident L5.end A1
  constraint horizontal L6
  constraint tangent L3 A0
  constraint concentric A2 A3
  constraint tangent L13 A2
  constraint coincident L9 A4.end
  constraint concentric A3 A4
  constraint concentric A3 A5
  measures "d1" distance of L0.end L1.end
  measures "d2" distance of L1.end L2.end
  measures "d4" distance of L4.end L5.end
  measures "d6" distance of L3 L13
  measures "d9" distance of A1 A2
  measures "d14" distance of A0 A3
extrude "Extrude1" add sketch "Sketch1" along normal mid plane 151 contours L4 L5 L6 L7 makes body 1
sketch "Sketch3" plane through (0, 0, 0) normal (0, 0, 1) x (-1, 0, 0)
  circle A0 centre (7, -45) radius 5
extrude "Extrude2" add sketch "Sketch3" along normal mid plane 175 bodies 1
sketch "Sketch4" plane through (0, 0, 0) normal (0, 0, 1) x (1, 0, 0)
  line L0 (-22.6192, 50) -> (-22.6192, 40)
  line L1 (-22.6192, 46.5) -> (-30.0211, 46.5)
  line L2 (-32.6192, 46.5) -> (-32.6192, 43.5) construction
  line L3 (-30.0211, 43.5) -> (-22.6192, 43.5)
  line L4 (-22.6192, 43.5) -> (-22.6192, 46.5)
  arc A0 (-30.0211, 46.5) -> (-30.0211, 43.5) centre (-32.6192, 45) ccw
  arc A1 (-30.0211, 43.5) -> (-30.0211, 46.5) centre (-32.6192, 45) ccw construction
  line L5 (-30.0211, 46.5) -> (-32.6192, 46.5) construction
  line L6 (-32.6192, 43.5) -> (-30.0211, 43.5) construction
  point P0 (-22.6192, 45)
  dimension "d20" = 6
  dimension "d22" = 10
  dimension "d30" = 3
  constraint midpoint L0 P0
  constraint horizontal L1
  constraint vertical L2
  constraint horizontal L3
  constraint vertical L4
  constraint coincident L0 L1.start
  constraint midpoint P0 L4
  constraint midpoint L2 A0.centre
  constraint concentric A0 A1
  constraint horizontal L5
  constraint horizontal L6
  measures "d20" diameter of A0
  measures "d22" distance of L0 A0.centre
  measures "d30" distance of L1 L3
extrude "Extrude3" add sketch "Sketch4" along normal mid plane 20 separate body makes body 2
sketch "Sketch6" plane through (0, 0, 0) normal (0, 0, 1) x (1, 0, 0)
  arc A0 (-30.0211, 46.5) -> (-30.0211, 43.5) centre (-32.6192, 45) ccw construction
  line L0 (-22.6192, 46.5) -> (-30.0211, 46.5)
  line L1 (-30.0211, 46.5) -> (-30.0211, 43.5)
  line L2 (-30.0211, 43.5) -> (-22.6192, 43.5)
  line L3 (-22.6192, 43.5) -> (-22.6192, 46.5)
  arc A1 (-30.0211, 46.5) -> (-30.0211, 43.5) centre (-32.6192, 45) ccw construction
  arc A2 (-30.0211, 43.5) -> (-30.0211, 46.5) centre (-32.6192, 45) ccw
  dimension "d27" = 10
  constraint concentric A0 A1
  constraint equal A0 A1
  constraint horizontal L0
  constraint vertical L1
  constraint horizontal L2
  constraint vertical L3
  constraint coincident A0.start L0.end
  constraint coincident A0.end L1.end
  constraint concentric A1 A2
  measures "d27" distance of A0.centre L3
extrude "Extrude4" cut sketch "Sketch6" along normal mid plane 10 contours L0 L2 L3 A2 bodies 2
